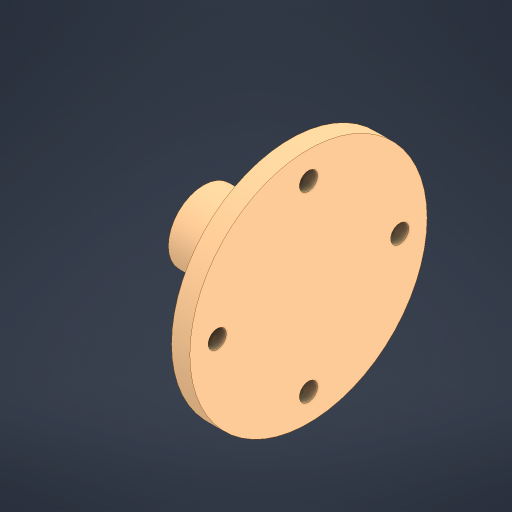
# Autodesk Inventor part: acople_stepper
Saved by Autodesk Inventor 2023.1 (Build 271208000, 208)
## iProperties
Created: 2022-10-28
Part Number: acople_stepper
Material: Generic
Document SubType Name: Modeling
Designer: amtat
Density: 1 g/cm^3
Appearance: Default
Author: amtat
Autodesk Inventor part; units mm, degrees
ref_plane "YZ Plane" through (0, 0, 0) normal (1, 0, 0) x (0, 1, 0)
ref_plane "XZ Plane" through (0, 0, 0) normal (0, 1, 0) x (-1, 0, 0)
ref_plane "XY Plane" through (0, 0, 0) normal (0, 0, 1) x (1, 0, 0)
sketch "Sketch1" plane through (0, 0, 0) normal (1, 0, 0) x (0, 1, 0)
  line L0 (0, 0) -> (2.5, 0)
  line L1 (2.5, 0) -> (2.5, -1.5)
  line L2 (2.5, -1.5) -> (2.5, 1.5)
  circle A0 centre (0, 0) radius 2.5
  line L3 (2.5, 1.5) -> (-2.5, 1.5)
  line L4 (-2.5, 1.5) -> (-2.5, -1.5)
  line L5 (-2.5, -1.5) -> (2.5, -1.5)
  circle A1 centre (0, 0) radius 5.5
  point P0 (-2, -1.5)
  point P1 (-2, 1.5)
  point P2 (2, 1.5)
  point P3 (2, -1.5)
  dimension "d0" = 2.5
  dimension "d1" = 1.5
  dimension "d2" = 3
  dimension "d3" = 5
  dimension "d4" = 3
  dimension "d5" = 11
  constraints: 12 end point, 2 coincident, 2 horizontal, 2 perpendicular, 1 centre point, 1 point on line, 3 other
  measures "d0" distance of L0.start L0.end
  measures "d1" distance of L0.end L1.end
  measures "d2" distance of L1.end L2.end
  measures "d3" distance of L2.end L3.end
  measures "d4" distance of L3.end L4.end
  measures "d5" diameter of A1
extrude "Extrusion1" add sketch "Sketch1" along normal blind 7 contours A0 L3 L2 | L1 L5 A0 | L3 A0 | A0 L5 | A0 L4 L3 | L5 L4 A0 | A1
sketch "Sketch2" plane through (7, 0, 0) normal (1, 0, 0) x (0, 0, -1)
  circle A0 centre (0, 0) radius 5.5 projected
  arc A1 (-1.5, -2) -> (1.5, -2) centre (0, 0) ccw projected
  line L0 (-1.5, -2) -> (-1.5, 2) projected
  arc A2 (1.5, 2) -> (-1.5, 2) centre (0, 0) ccw projected
  line L1 (1.5, 2) -> (1.5, -2) projected
  circle A3 centre (0, 10) radius 0.5
  circle A4 centre (10, 0) radius 0.5
  circle A5 centre (0, -10) radius 0.5
  circle A6 centre (-10, 0) radius 0.5
  circle A7 centre (0, 0) radius 13
  arc A8 (-9.9875, 0.4998) -> (0.4998, -9.9875) centre (0, 0) ccw
  arc A9 (9.9875, -0.4998) -> (-0.4998, 9.9875) centre (0, 0) ccw
  dimension "d9" = 1
  dimension "d10" = 1
  dimension "d11" = 1
  dimension "d12" = 1
  dimension "d13" = 26
  constraints: 8 point on circle, 3 centre point, 2 coincident, 12 other
  measures "d13" diameter of A7
extrude "Extrusion2" add sketch "Sketch2" against normal blind 2 contours A7
sketch "Sketch3" plane through (7, 0, 0) normal (1, 0, 0) x (0, 0, -1)
  circle A0 centre (0, -10) radius 0.5 projected
  circle A1 centre (0, 10) radius 0.5 projected
  circle A2 centre (10, 0) radius 0.5 projected
  circle A3 centre (-10, 0) radius 0.5 projected
  circle A4 centre (0, 0) radius 13 projected
  arc A5 (-1.5, -2) -> (1.5, -2) centre (0, 0) ccw projected
  line L0 (-1.5, -2) -> (-1.5, 2) projected
  arc A6 (1.5, 2) -> (-1.5, 2) centre (0, 0) ccw projected
  line L1 (1.5, 2) -> (1.5, -2) projected
  circle A7 centre (0, 10) radius 1
  circle A8 centre (-10, 0) radius 0.5 projected
  circle A9 centre (-10, 0) radius 1
  circle A10 centre (10, 0) radius 0.5 projected
  circle A11 centre (10, 0) radius 1
  circle A12 centre (0, -10) radius 1
  dimension "d17" = 2
  dimension "d18" = 2
  dimension "d19" = 2
  dimension "d20" = 2
  constraints: 4 centre point, 4 coincident
  measures "d17" diameter of A7
  measures "d18" diameter of A9
  measures "d19" diameter of A11
  measures "d20" diameter of A12
extrude "Extrusion3" cut sketch "Sketch3" against normal blind 10 contours A0 | A1 | A3 | A7 | A9 | A11 | A12
sketch "Sketch4" plane through (7, 0, 0) normal (1, 0, 0) x (0, 0, -1)
  arc A0 (-1.5, -2) -> (1.5, -2) centre (0, 0) ccw projected
  line L0 (1.5, 2) -> (1.5, -2) projected
  arc A1 (1.5, 2) -> (-1.5, 2) centre (0, 0) ccw projected
  line L1 (-1.5, -2) -> (-1.5, 2) projected
extrude "Extrusion4" add sketch "Sketch4" against normal blind 7
sketch "Sketch5" plane through (0, 0, 0) normal (-1, 0, 0) x (0, 0, 1)
  circle A0 centre (0, 0) radius 5.5 projected
extrude "Extrusion5" cut sketch "Sketch5" against normal blind 5
sketch "Sketch6" plane through (5, 0, 0) normal (-1, 0, 0) x (0, 0, 1)
  circle A0 centre (0, 0) radius 3.85
  dimension "d27" = 7.7
  constraints: 1 centre point, 1 coincident
  measures "d27" diameter of A0
extrude "Extrusion6" add sketch "Sketch6" along normal blind 9.5
fillet "Fillet2" radius 1 1 edges at (5, 0, -3.85)
body "Solid1"
